Autodesk Inventor part; units mm, degrees
(part 2 of 2)
  line L353 (186.3853, -129.3179) -> (186.3853, -143.3229)
  line L354 (186.3853, -143.3229) -> (172.3803, -143.3229)
  line L355 (172.3803, -143.3229) -> (172.3803, -129.3179)
  line L356 (172.3803, -129.3179) -> (186.3853, -143.3229) construction
  line L357 (186.3853, -129.3179) -> (172.3803, -143.3229) construction
  line L358 (180.9186, -148.2929) -> (194.9236, -148.2929)
  line L359 (194.9236, -148.2929) -> (194.9236, -162.2979)
  line L360 (194.9236, -162.2979) -> (180.9186, -162.2979)
  line L361 (180.9186, -162.2979) -> (180.9186, -148.2929)
  line L362 (180.9186, -148.2929) -> (194.9236, -162.2979) construction
  line L363 (194.9236, -148.2929) -> (180.9186, -162.2979) construction
  line L364 (191.4303, -129.3179) -> (205.4353, -129.3179)
  line L365 (205.4353, -129.3179) -> (205.4353, -143.3229)
  line L366 (205.4353, -143.3229) -> (191.4303, -143.3229)
  line L367 (191.4303, -143.3229) -> (191.4303, -129.3179)
  line L368 (191.4303, -129.3179) -> (205.4353, -143.3229) construction
  line L369 (205.4353, -129.3179) -> (191.4303, -143.3229) construction
  line L370 (200.8283, -110.2679) -> (214.8333, -110.2679)
  line L371 (214.8333, -110.2679) -> (214.8333, -124.2729)
  line L372 (214.8333, -124.2729) -> (200.8283, -124.2729)
  line L373 (200.8283, -124.2729) -> (200.8283, -110.2679)
  line L374 (200.8283, -110.2679) -> (214.8333, -124.2729) construction
  line L375 (214.8333, -110.2679) -> (200.8283, -124.2729) construction
  line L376 (196.0023, -91.2179) -> (210.0073, -91.2179)
  line L377 (210.0073, -91.2179) -> (210.0073, -105.2229)
  line L378 (210.0073, -105.2229) -> (196.0023, -105.2229)
  line L379 (196.0023, -105.2229) -> (196.0023, -91.2179)
  line L380 (196.0023, -91.2179) -> (210.0073, -105.2229) construction
  line L381 (210.0073, -91.2179) -> (196.0023, -105.2229) construction
  line L382 (215.0523, -91.2179) -> (229.0573, -91.2179)
  line L383 (229.0573, -91.2179) -> (229.0573, -105.2229)
  line L384 (229.0573, -105.2229) -> (215.0523, -105.2229)
  line L385 (215.0523, -105.2229) -> (215.0523, -91.2179)
  line L386 (215.0523, -91.2179) -> (229.0573, -105.2229) construction
  line L387 (229.0573, -91.2179) -> (215.0523, -105.2229) construction
  line L388 (219.8783, -110.2679) -> (233.8833, -110.2679)
  line L389 (233.8833, -110.2679) -> (233.8833, -124.2729)
  line L390 (233.8833, -124.2729) -> (219.8783, -124.2729)
  line L391 (219.8783, -124.2729) -> (219.8783, -110.2679)
  line L392 (219.8783, -110.2679) -> (233.8833, -124.2729) construction
  line L393 (233.8833, -110.2679) -> (219.8783, -124.2729) construction
  line L394 (210.4803, -129.3179) -> (224.4853, -129.3179)
  line L395 (224.4853, -129.3179) -> (224.4853, -143.3229)
  line L396 (224.4853, -143.3229) -> (210.4803, -143.3229)
  line L397 (210.4803, -143.3229) -> (210.4803, -129.3179)
  line L398 (210.4803, -129.3179) -> (224.4853, -143.3229) construction
  line L399 (224.4853, -129.3179) -> (210.4803, -143.3229) construction
  line L400 (274.4883, -43.5111) -> (288.4933, -43.5111) construction
  line L401 (288.4933, -43.5111) -> (288.4933, -57.5161) construction
  line L402 (288.4933, -57.5161) -> (274.4883, -57.5161) construction
  line L403 (274.4883, -57.5161) -> (274.4883, -43.5111) construction
  line L404 (274.4883, -43.5111) -> (288.4933, -57.5161) construction
  line L405 (288.4933, -43.5111) -> (274.4883, -57.5161) construction
  line L406 (281.8543, -72.1679) -> (295.8593, -72.1679) construction
  line L407 (295.8593, -72.1679) -> (295.8593, -86.1729) construction
  line L408 (295.8593, -86.1729) -> (281.8543, -86.1729) construction
  line L409 (281.8543, -86.1729) -> (281.8543, -72.1679) construction
  line L410 (281.8543, -72.1679) -> (295.8593, -86.1729) construction
  line L411 (295.8593, -72.1679) -> (281.8543, -86.1729) construction
  line L412 (272.2023, -91.2179) -> (286.2073, -91.2179) construction
  line L413 (286.2073, -91.2179) -> (286.2073, -105.2229) construction
  line L414 (286.2073, -105.2229) -> (272.2023, -105.2229) construction
  line L415 (272.2023, -105.2229) -> (272.2023, -91.2179) construction
  line L416 (272.2023, -91.2179) -> (286.2073, -105.2229) construction
  line L417 (286.2073, -91.2179) -> (272.2023, -105.2229) construction
  line L418 (277.2823, -110.2679) -> (291.2873, -110.2679) construction
  line L419 (291.2873, -110.2679) -> (291.2873, -124.2729) construction
  line L420 (291.2873, -124.2729) -> (277.2823, -124.2729) construction
  line L421 (277.2823, -124.2729) -> (277.2823, -110.2679) construction
  line L422 (277.2823, -110.2679) -> (291.2873, -124.2729) construction
  line L423 (291.2873, -110.2679) -> (277.2823, -124.2729) construction
  line L424 (267.6303, -129.3179) -> (281.6353, -129.3179) construction
  line L425 (281.6353, -129.3179) -> (281.6353, -143.3229) construction
  line L426 (281.6353, -143.3229) -> (267.6303, -143.3229) construction
  line L427 (267.6303, -143.3229) -> (267.6303, -129.3179) construction
  line L428 (267.6303, -129.3179) -> (281.6353, -143.3229) construction
  line L429 (281.6353, -129.3179) -> (267.6303, -143.3229) construction
  line L430 (279.0603, -148.3679) -> (293.0653, -148.3679) construction
  line L431 (293.0653, -148.3679) -> (293.0653, -162.3729) construction
  line L432 (293.0653, -162.3729) -> (279.0603, -162.3729) construction
  line L433 (279.0603, -162.3729) -> (279.0603, -148.3679) construction
  line L434 (279.0603, -148.3679) -> (293.0653, -162.3729) construction
  line L435 (293.0653, -148.3679) -> (279.0603, -162.3729) construction
  line L436 (269.5528, -40) -> (269.5528, -64.842) construction
  line L437 (269.5528, -64.842) -> (279.3318, -64.842) construction
  line L438 (279.3318, -64.842) -> (279.3318, -88.6954) construction
  line L439 (279.3318, -88.6954) -> (269.6798, -88.6954) construction
  line L440 (269.6798, -88.6954) -> (269.6798, -107.7454) construction
  line L441 (269.6798, -107.7454) -> (274.7598, -107.7454) construction
  line L442 (265.1048, -126.7954) -> (265.1048, -151.6615) construction
  line L443 (265.1048, -151.6615) -> (275.5314, -151.6615) construction
  line L444 (275.5314, -151.6615) -> (275.5314, -165) construction
  line L445 (265, -160) -> (275.5314, -160) construction
  line L446 (286.0628, -155.3704) -> (275.5314, -155.3704) construction
  line L447 (265, -160) -> (265, -151.6615) construction
  line L448 (269.0122, -143.3229) -> (269.0122, -151.6615) construction
  line L449 (262.5793, -140.2954) -> (265.1048, -140.2954) construction
  line L450 (265.1048, -140.2954) -> (267.6303, -140.2954) construction
  line L451 (273.1318, -105.2229) -> (273.1318, -107.7454) construction
  line L452 (271.7643, -110.2679) -> (271.7643, -107.7454) construction
  line L453 (267.1573, -99.7852) -> (269.6798, -99.7852) construction
  line L454 (269.6798, -99.7852) -> (272.2023, -99.7852) construction
  line L455 (273.1318, -91.2179) -> (273.1318, -88.6954) construction
  line L456 (273.1318, -88.6954) -> (273.1318, -86.1729) construction
  line L457 (276.8093, -76.5209) -> (279.3318, -76.5209) construction
  line L458 (279.3318, -76.5209) -> (281.8543, -76.5209) construction
  line L459 (276.0401, -72.1679) -> (276.0401, -64.842) construction
  line L460 (276.0401, -64.842) -> (276.0401, -57.5161) construction
  line L461 (264.6173, -51.0859) -> (269.5528, -51.0859) construction
  line L462 (269.5528, -51.0859) -> (274.4883, -51.0859) construction
  line L463 (274.7598, -107.7454) -> (274.7598, -126.7954) construction
  line L464 (272.2373, -121.2454) -> (274.7598, -121.2454) construction
  line L465 (274.7598, -121.2454) -> (277.2823, -121.2454) construction
  line L466 (265.1048, -126.7954) -> (274.7598, -126.7954) construction
  line L467 (270.2657, -124.2729) -> (270.2657, -126.7954) construction
  line L468 (270.2657, -126.7954) -> (270.2657, -129.3179) construction
  line L469 (269.4028, -40) -> (269.4028, -64.992)
  line L470 (269.4028, -64.992) -> (279.1818, -64.992)
  line L471 (279.1818, -64.992) -> (279.1818, -88.5454)
  line L472 (279.1818, -88.5454) -> (269.5298, -88.5454)
  line L473 (269.5298, -88.5454) -> (269.5298, -107.8954)
  line L474 (269.5298, -107.8954) -> (274.6098, -107.8954)
  line L475 (274.6098, -107.8954) -> (274.6098, -126.6454)
  line L476 (274.6098, -126.6454) -> (264.9548, -126.6454)
  line L477 (264.9548, -126.6454) -> (264.9548, -151.8115)
  line L478 (264.9548, -151.8115) -> (275.3814, -151.8115)
  line L479 (275.3814, -151.8115) -> (275.3814, -165)
  line L480 (275.3814, -165) -> (40, -165)
  line L481 (40, -165) -> (40, -40)
  line L482 (40, -40) -> (269.4028, -40)
  circle A409 centre (45, -127) radius 3.25
  circle A410 centre (45, -64.8616) radius 3.25
  line L483 (172.0148, -58.6601) -> (214.7648, -58.6601)
  line L484 (214.7648, -58.6601) -> (214.7648, -65.1601)
  line L485 (214.7648, -65.1601) -> (172.0148, -65.1601)
  line L486 (172.0148, -65.1601) -> (172.0148, -58.6601)
  circle A411 centre (155, -64.8616) radius 3.25
  circle A412 centre (265, -64.8616) radius 3.25
  point P0 (0, 0)
  point P1 (274.7598, -117.2704)
  point P2 (46.7679, -124.2729)
  point P3 (46.1423, -123.9574)
  dimension "d0" = 6.5
  dimension "d1" = 14.005
  dimension "d2" = 14.005
  dimension "d3" = 14.005
  dimension "d4" = 14.005
  dimension "d5" = 14.005
  dimension "d6" = 14.005
  dimension "d7" = 14.005
  dimension "d8" = 14.005
  dimension "d9" = 14.005
  dimension "d10" = 14.005
  dimension "d11" = 14.005
  dimension "d12" = 14.005
  dimension "d13" = 14.005
  dimension "d14" = 14.005
  dimension "d15" = 14.005
  dimension "d16" = 14.005
  dimension "d17" = 14.005
  dimension "d18" = 14.005
  dimension "d19" = 14.005
  dimension "d20" = 14.005
  dimension "d21" = 14.005
  dimension "d22" = 14.005
  dimension "d23" = 14.005
  dimension "d24" = 14.005
  dimension "d25" = 14.005
  dimension "d26" = 14.005
  dimension "d27" = 14.005
  dimension "d28" = 14.005
  dimension "d29" = 14.005
  dimension "d30" = 14.005
  dimension "d31" = 14.005
  dimension "d32" = 14.005
  dimension "d33" = 14.005
  dimension "d34" = 14.005
  dimension "d35" = 14.005
  dimension "d36" = 14.005
  dimension "d37" = 14.005
  dimension "d38" = 14.005
  dimension "d39" = 14.005
  dimension "d40" = 14.005
  dimension "d41" = 14.005
  dimension "d42" = 14.005
  dimension "d43" = 14.005
  dimension "d44" = 14.005
  dimension "d45" = 14.005
  dimension "d46" = 14.005
  dimension "d47" = 14.005
  dimension "d48" = 14.005
  dimension "d49" = 14.005
  dimension "d50" = 14.005
  dimension "d51" = 14.005
  dimension "d52" = 14.005
  dimension "d53" = 14.005
  dimension "d54" = 14.005
  dimension "d55" = 14.005
  dimension "d56" = 14.005
  dimension "d57" = 14.005
  dimension "d58" = 14.005
  dimension "d59" = 14.005
  dimension "d60" = 14.005
  dimension "d61" = 14.005
  dimension "d62" = 14.005
  dimension "d63" = 14.005
  constraints: 870 end point, 132 parallel, 129 midpoint, 92 perpendicular, 67 horizontal, 47 point on line, 11 equal length, 7 coincident, 6 centre point, 5 equal radius, 3 collinear, 2 vertical
  measures "d0" diameter of A407
  measures "d1" distance of L54.end L53.end
  measures "d2" distance of L53.end L52.end
  measures "d3" distance of L59.end L60.end
  measures "d4" distance of L58.end L59.end
  measures "d5" distance of L65.end L66.end
  measures "d6" distance of L64.end L65.end
  measures "d7" distance of L71.end L72.end
  measures "d8" distance of L70.end L71.end
  measures "d9" distance of L77.end L78.end
  measures "d10" distance of L76.end L77.end
  measures "d11" distance of L83.end L84.end
  measures "d12" distance of L82.end L83.end
  measures "d13" distance of L89.end L90.end
  measures "d14" distance of L88.end L89.end
  measures "d15" distance of L95.end L96.end
  measures "d16" distance of L94.end L95.end
  measures "d17" distance of L101.end L102.end
  measures "d18" distance of L100.end L101.end
  measures "d19" distance of L107.end L108.end
  measures "d20" distance of L106.end L107.end
  measures "d21" distance of L113.end L114.end
  measures "d22" distance of L112.end L113.end
  measures "d23" distance of L119.end L120.end
  measures "d24" distance of L118.end L119.end
  measures "d25" distance of L125.end L126.end
  measures "d26" distance of L124.end L125.end
  measures "d27" distance of L131.end L132.end
  measures "d28" distance of L130.end L131.end
  measures "d29" distance of L137.end L138.end
  measures "d30" distance of L136.end L137.end
  measures "d31" distance of L143.end L144.end
  measures "d32" distance of L142.end L143.end
  measures "d33" distance of L149.end L150.end
  measures "d34" distance of L148.end L149.end
  measures "d35" distance of L155.end L156.end
  measures "d36" distance of L154.end L155.end
  measures "d37" distance of L161.end L162.end
  measures "d38" distance of L160.end L161.end
  measures "d39" distance of L167.end L168.end
  measures "d40" distance of L166.end L167.end
  measures "d41" distance of L173.end L174.end
  measures "d42" distance of L172.end L173.end
  measures "d43" distance of L179.end L180.end
  measures "d44" distance of L178.end L179.end
  measures "d45" distance of L185.end L186.end
  measures "d46" distance of L184.end L185.end
  measures "d47" distance of L191.end L192.end
  measures "d48" distance of L190.end L191.end
  measures "d49" distance of L197.end L198.end
  measures "d50" distance of L196.end L197.end
  measures "d51" distance of L203.end L204.end
  measures "d52" distance of L202.end L203.end
  measures "d53" distance of L209.end L210.end
  measures "d54" distance of L208.end L209.end
  measures "d55" distance of L215.end L216.end
  measures "d56" distance of L214.end L215.end
  measures "d57" distance of L221.end L222.end
  measures "d58" distance of L220.end L221.end
  measures "d59" distance of L227.end L228.end
  measures "d60" distance of L226.end L227.end
  measures "d61" distance of L233.end L234.end
  measures "d62" distance of L232.end L233.end
  measures "d63" distance of L239.end L240.end
extrude "Extrusion3" add sketch "Sketch1" along normal blind 0.5
sketch "Sketch3" plane through (0, 0, 0.5) normal (0, 0, 1) x (1, 0, 0)
  line L0 (40, -40) -> (40, -165) projected
  line L1 (40, -165) -> (275.3814, -165) projected
  line L2 (275.3814, -165) -> (275.3814, -151.8115) projected
  line L3 (275.3814, -151.8115) -> (264.9548, -151.8115) projected
  line L4 (264.9548, -151.8115) -> (264.9548, -126.6454) projected
  line L5 (264.9548, -126.6454) -> (274.6098, -126.6454) projected
  line L6 (274.6098, -126.6454) -> (274.6098, -107.8954) projected
  line L7 (274.6098, -107.8954) -> (269.5298, -107.8954) projected
  line L8 (269.5298, -107.8954) -> (269.5298, -88.5454) projected
  line L9 (269.5298, -88.5454) -> (279.1818, -88.5454) projected
  line L10 (279.1818, -88.5454) -> (279.1818, -64.992) projected
  line L11 (279.1818, -64.992) -> (269.4028, -64.992) projected
  line L12 (269.4028, -64.992) -> (269.4028, -40) projected
  line L13 (269.4028, -40) -> (40, -40) projected
  circle A0 centre (155, -160) radius 3.25 projected
  circle A1 centre (265, -160) radius 3.25 projected
  circle A2 centre (45, -64.8616) radius 3.25 projected
  circle A3 centre (155, -64.8616) radius 3.25 projected
  circle A4 centre (265, -64.8616) radius 3.25 projected
  line L14 (172.0148, -58.6601) -> (214.7648, -58.6601) projected
  line L15 (214.7648, -58.6601) -> (214.7648, -65.1601) projected
  line L16 (214.7648, -65.1601) -> (172.0148, -65.1601) projected
  line L17 (172.0148, -65.1601) -> (172.0148, -58.6601) projected
  line L18 (210.4803, -129.3179) -> (224.4853, -129.3179) projected
  line L19 (224.4853, -129.3179) -> (224.4853, -143.3229) projected
  line L20 (224.4853, -143.3229) -> (210.4803, -143.3229) projected
  line L21 (210.4803, -143.3229) -> (210.4803, -129.3179) projected
  line L22 (219.8783, -110.2679) -> (233.8833, -110.2679) projected
  line L23 (233.8833, -110.2679) -> (233.8833, -124.2729) projected
  line L24 (233.8833, -124.2729) -> (219.8783, -124.2729) projected
  line L25 (219.8783, -124.2729) -> (219.8783, -110.2679) projected
  line L26 (215.0523, -91.2179) -> (229.0573, -91.2179) projected
  line L27 (229.0573, -91.2179) -> (229.0573, -105.2229) projected
  line L28 (229.0573, -105.2229) -> (215.0523, -105.2229) projected
  line L29 (215.0523, -105.2229) -> (215.0523, -91.2179) projected
  line L30 (196.0023, -91.2179) -> (210.0073, -91.2179) projected
  line L31 (210.0073, -91.2179) -> (210.0073, -105.2229) projected
  line L32 (210.0073, -105.2229) -> (196.0023, -105.2229) projected
  line L33 (196.0023, -105.2229) -> (196.0023, -91.2179) projected
  line L34 (200.8283, -110.2679) -> (214.8333, -110.2679) projected
  line L35 (214.8333, -110.2679) -> (214.8333, -124.2729) projected
  line L36 (214.8333, -124.2729) -> (200.8283, -124.2729) projected
  line L37 (200.8283, -124.2729) -> (200.8283, -110.2679) projected
  line L38 (191.4303, -129.3179) -> (205.4353, -129.3179) projected
  line L39 (205.4353, -129.3179) -> (205.4353, -143.3229) projected
  line L40 (205.4353, -143.3229) -> (191.4303, -143.3229) projected
  line L41 (191.4303, -143.3229) -> (191.4303, -129.3179) projected
  line L42 (180.9186, -148.2929) -> (194.9236, -148.2929) projected
  line L43 (194.9236, -148.2929) -> (194.9236, -162.2979) projected
  line L44 (194.9236, -162.2979) -> (180.9186, -162.2979) projected
  line L45 (180.9186, -162.2979) -> (180.9186, -148.2929) projected
  line L46 (172.3803, -129.3179) -> (186.3853, -129.3179) projected
  line L47 (186.3853, -129.3179) -> (186.3853, -143.3229) projected
  line L48 (186.3853, -143.3229) -> (172.3803, -143.3229) projected
  line L49 (172.3803, -143.3229) -> (172.3803, -129.3179) projected
  line L50 (181.7783, -110.2679) -> (195.7833, -110.2679) projected
  line L51 (195.7833, -110.2679) -> (195.7833, -124.2729) projected
  line L52 (195.7833, -124.2729) -> (181.7783, -124.2729) projected
  line L53 (181.7783, -124.2729) -> (181.7783, -110.2679) projected
  line L54 (176.9523, -91.2179) -> (190.9573, -91.2179) projected
  line L55 (190.9573, -91.2179) -> (190.9573, -105.2229) projected
  line L56 (190.9573, -105.2229) -> (176.9523, -105.2229) projected
  line L57 (176.9523, -105.2229) -> (176.9523, -91.2179) projected
  line L58 (162.7283, -110.2679) -> (176.7333, -110.2679) projected
  line L59 (176.7333, -110.2679) -> (176.7333, -124.2729) projected
  line L60 (176.7333, -124.2729) -> (162.7283, -124.2729) projected
  line L61 (162.7283, -124.2729) -> (162.7283, -110.2679) projected
  line L62 (157.9023, -91.2967) -> (171.9073, -91.2967) projected
  line L63 (171.9073, -91.2967) -> (171.9073, -105.3017) projected
  line L64 (171.9073, -105.3017) -> (157.9023, -105.3017) projected
  line L65 (157.9023, -105.3017) -> (157.9023, -91.2967) projected
  line L66 (153.3303, -129.3179) -> (167.3353, -129.3179) projected
  line L67 (167.3353, -129.3179) -> (167.3353, -143.3229) projected
  line L68 (167.3353, -143.3229) -> (153.3303, -143.3229) projected
  line L69 (153.3303, -143.3229) -> (153.3303, -129.3179) projected
  line L70 (134.2803, -129.3179) -> (148.2853, -129.3179) projected
  line L71 (148.2853, -129.3179) -> (148.2853, -143.3229) projected
  line L72 (148.2853, -143.3229) -> (134.2803, -143.3229) projected
  line L73 (134.2803, -143.3229) -> (134.2803, -129.3179) projected
  line L74 (143.6783, -110.2679) -> (157.6833, -110.2679) projected
  line L75 (157.6833, -110.2679) -> (157.6833, -124.2729) projected
  line L76 (157.6833, -124.2729) -> (143.6783, -124.2729) projected
  line L77 (143.6783, -124.2729) -> (143.6783, -110.2679) projected
  line L78 (138.8523, -91.2179) -> (152.8573, -91.2179) projected
  line L79 (152.8573, -91.2179) -> (152.8573, -105.2229) projected
  line L80 (152.8573, -105.2229) -> (138.8523, -105.2229) projected
  line L81 (138.8523, -105.2229) -> (138.8523, -91.2179) projected
  line L82 (119.8023, -91.2179) -> (133.8073, -91.2179) projected
  line L83 (133.8073, -91.2179) -> (133.8073, -105.2229) projected
  line L84 (133.8073, -105.2229) -> (119.8023, -105.2229) projected
  line L85 (119.8023, -105.2229) -> (119.8023, -91.2179) projected
  line L86 (124.6283, -110.2679) -> (138.6333, -110.2679) projected
  line L87 (138.6333, -110.2679) -> (138.6333, -124.2729) projected
  line L88 (138.6333, -124.2729) -> (124.6283, -124.2729) projected
  line L89 (124.6283, -124.2729) -> (124.6283, -110.2679) projected
  line L90 (115.2303, -129.3179) -> (129.2353, -129.3179) projected
  line L91 (129.2353, -129.3179) -> (129.2353, -143.3229) projected
  line L92 (129.2353, -143.3229) -> (115.2303, -143.3229) projected
  line L93 (115.2303, -143.3229) -> (115.2303, -129.3179) projected
  line L94 (96.1803, -129.3179) -> (110.1853, -129.3179) projected
  line L95 (110.1853, -129.3179) -> (110.1853, -143.3229) projected
  line L96 (110.1853, -143.3229) -> (96.1803, -143.3229) projected
  line L97 (96.1803, -143.3229) -> (96.1803, -129.3179) projected
  line L98 (105.5783, -110.2679) -> (119.5833, -110.2679) projected
  line L99 (119.5833, -110.2679) -> (119.5833, -124.2729) projected
  line L100 (119.5833, -124.2729) -> (105.5783, -124.2729) projected
  line L101 (105.5783, -124.2729) -> (105.5783, -110.2679) projected
  line L102 (100.7523, -91.2179) -> (114.7573, -91.2179) projected
  line L103 (114.7573, -91.2179) -> (114.7573, -105.2229) projected
  line L104 (114.7573, -105.2229) -> (100.7523, -105.2229) projected
  line L105 (100.7523, -105.2229) -> (100.7523, -91.2179) projected
  line L106 (86.5283, -110.2679) -> (100.5333, -110.2679) projected
  line L107 (100.5333, -110.2679) -> (100.5333, -124.2729) projected
  line L108 (100.5333, -124.2729) -> (86.5283, -124.2729) projected
  line L109 (86.5283, -124.2729) -> (86.5283, -110.2679) projected
  line L110 (77.1303, -129.3179) -> (91.1353, -129.3179) projected
  line L111 (91.1353, -129.3179) -> (91.1353, -143.3229) projected
  line L112 (91.1353, -143.3229) -> (77.1303, -143.3229) projected
  line L113 (77.1303, -143.3229) -> (77.1303, -129.3179) projected
  line L114 (83.7343, -148.3679) -> (97.7393, -148.3679) projected
  line L115 (97.7393, -148.3679) -> (97.7393, -162.3729) projected
  line L116 (97.7393, -162.3729) -> (83.7343, -162.3729) projected
  line L117 (83.7343, -162.3729) -> (83.7343, -148.3679) projected
  line L118 (59.8583, -148.3679) -> (73.8633, -148.3679) projected
  line L119 (73.8633, -148.3679) -> (73.8633, -162.3729) projected
  line L120 (73.8633, -162.3729) -> (59.8583, -162.3729) projected
  line L121 (59.8583, -162.3729) -> (59.8583, -148.3679) projected
  line L122 (50.9683, -129.3179) -> (64.9733, -129.3179) projected
  line L123 (64.9733, -129.3179) -> (64.9733, -143.3229) projected
  line L124 (64.9733, -143.3229) -> (50.9683, -143.3229) projected
  line L125 (50.9683, -143.3229) -> (50.9683, -129.3179) projected
  line L126 (67.4783, -110.2679) -> (81.4833, -110.2679) projected
  line L127 (81.4833, -110.2679) -> (81.4833, -124.2729) projected
  line L128 (81.4833, -124.2729) -> (67.4783, -124.2729) projected
  line L129 (67.4783, -124.2729) -> (67.4783, -110.2679) projected
  line L130 (81.7023, -91.2179) -> (95.7073, -91.2179) projected
  line L131 (95.7073, -91.2179) -> (95.7073, -105.2229) projected
  line L132 (95.7073, -105.2229) -> (81.7023, -105.2229) projected
  line L133 (81.7023, -105.2229) -> (81.7023, -91.2179) projected
  line L134 (53.2543, -91.2179) -> (67.2593, -91.2179) projected
  line L135 (67.2593, -91.2179) -> (67.2593, -105.2229) projected
  line L136 (67.2593, -105.2229) -> (53.2543, -105.2229) projected
  line L137 (53.2543, -105.2229) -> (53.2543, -91.2179) projected
  line L138 (48.5263, -72.1679) -> (62.5313, -72.1679) projected
  line L139 (62.5313, -72.1679) -> (62.5313, -86.1729) projected
  line L140 (62.5313, -86.1729) -> (48.5263, -86.1729) projected
  line L141 (48.5263, -86.1729) -> (48.5263, -72.1679) projected
  line L142 (72.3043, -72.1679) -> (86.3093, -72.1679) projected
  line L143 (86.3093, -72.1679) -> (86.3093, -86.1729) projected
  line L144 (86.3093, -86.1729) -> (72.3043, -86.1729) projected
  line L145 (72.3043, -86.1729) -> (72.3043, -72.1679) projected
  line L146 (91.3543, -72.1679) -> (105.3593, -72.1679) projected
  line L147 (105.3593, -72.1679) -> (105.3593, -86.1729) projected
  line L148 (105.3593, -86.1729) -> (91.3543, -86.1729) projected
  line L149 (91.3543, -86.1729) -> (91.3543, -72.1679) projected
  line L150 (110.4043, -72.1679) -> (124.4093, -72.1679) projected
  line L151 (124.4093, -72.1679) -> (124.4093, -86.1729) projected
  line L152 (124.4093, -86.1729) -> (110.4043, -86.1729) projected
  line L153 (110.4043, -86.1729) -> (110.4043, -72.1679) projected
  line L154 (129.4543, -72.1679) -> (143.4593, -72.1679) projected
  line L155 (143.4593, -72.1679) -> (143.4593, -86.1729) projected
  line L156 (143.4593, -86.1729) -> (129.4543, -86.1729) projected
  line L157 (129.4543, -86.1729) -> (129.4543, -72.1679) projected
  line L158 (148.5043, -72.1679) -> (162.5093, -72.1679) projected
  line L159 (162.5093, -72.1679) -> (162.5093, -86.1729) projected
  line L160 (162.5093, -86.1729) -> (148.5043, -86.1729) projected
  line L161 (148.5043, -86.1729) -> (148.5043, -72.1679) projected
  line L162 (167.5543, -72.1679) -> (181.5593, -72.1679) projected
  line L163 (181.5593, -72.1679) -> (181.5593, -86.1729) projected
  line L164 (181.5593, -86.1729) -> (167.5543, -86.1729) projected
  line L165 (167.5543, -86.1729) -> (167.5543, -72.1679) projected
  line L166 (186.6043, -72.1679) -> (200.6093, -72.1679) projected
  line L167 (200.6093, -72.1679) -> (200.6093, -86.1729) projected
  line L168 (200.6093, -86.1729) -> (186.6043, -86.1729) projected
  line L169 (186.6043, -86.1729) -> (186.6043, -72.1679) projected
  line L170 (205.6543, -72.1679) -> (219.6593, -72.1679) projected
  line L171 (219.6593, -72.1679) -> (219.6593, -86.1729) projected
  line L172 (219.6593, -86.1729) -> (205.6543, -86.1729) projected
  line L173 (205.6543, -86.1729) -> (205.6543, -72.1679) projected
  line L174 (224.7043, -72.1679) -> (238.7093, -72.1679) projected
  line L175 (238.7093, -72.1679) -> (238.7093, -86.1729) projected
  line L176 (238.7093, -86.1729) -> (224.7043, -86.1729) projected
  line L177 (224.7043, -86.1729) -> (224.7043, -72.1679) projected
  line L178 (243.7543, -72.1679) -> (257.7593, -72.1679) projected
  line L179 (257.7593, -72.1679) -> (257.7593, -86.1729) projected
  line L180 (257.7593, -86.1729) -> (243.7543, -86.1729) projected
  line L181 (243.7543, -86.1729) -> (243.7543, -72.1679) projected
  line L182 (234.1023, -91.2179) -> (248.1073, -91.2179) projected
  line L183 (248.1073, -91.2179) -> (248.1073, -105.2229) projected
  line L184 (248.1073, -105.2229) -> (234.1023, -105.2229) projected
  line L185 (234.1023, -105.2229) -> (234.1023, -91.2179) projected
  line L186 (238.9283, -110.2679) -> (252.9333, -110.2679) projected
  line L187 (252.9333, -110.2679) -> (252.9333, -124.2729) projected
  line L188 (252.9333, -124.2729) -> (238.9283, -124.2729) projected
  line L189 (238.9283, -124.2729) -> (238.9283, -110.2679) projected
  line L190 (229.5343, -129.3199) -> (243.5393, -129.3199) projected
  line L191 (243.5393, -129.3199) -> (243.5393, -143.3249) projected
  line L192 (243.5393, -143.3249) -> (229.5343, -143.3249) projected
  line L193 (229.5343, -143.3249) -> (229.5343, -129.3199) projected
  line L194 (248.5743, -129.3399) -> (262.5793, -129.3399) projected
  line L195 (262.5793, -129.3399) -> (262.5793, -143.3449) projected
  line L196 (262.5793, -143.3449) -> (248.5743, -143.3449) projected
  line L197 (248.5743, -143.3449) -> (248.5743, -129.3399) projected
  line L198 (258.2323, -110.2679) -> (272.2373, -110.2679) projected
  line L199 (272.2373, -110.2679) -> (272.2373, -124.2729) projected
  line L200 (272.2373, -124.2729) -> (258.2323, -124.2729) projected
  line L201 (258.2323, -124.2729) -> (258.2323, -110.2679) projected
  line L202 (253.1523, -91.2179) -> (267.1573, -91.2179) projected
  line L203 (267.1573, -91.2179) -> (267.1573, -105.2229) projected
  line L204 (267.1573, -105.2229) -> (253.1523, -105.2229) projected
  line L205 (253.1523, -105.2229) -> (253.1523, -91.2179) projected
  line L206 (262.8043, -72.1679) -> (276.8093, -72.1679) projected
  line L207 (276.8093, -72.1679) -> (276.8093, -86.1729) projected
  line L208 (276.8093, -86.1729) -> (262.8043, -86.1729) projected
  line L209 (262.8043, -86.1729) -> (262.8043, -72.1679) projected
  line L210 (250.6123, -43.5111) -> (264.6173, -43.5111) projected
  line L211 (264.6173, -43.5111) -> (264.6173, -57.5161) projected
  line L212 (264.6173, -57.5161) -> (250.6123, -57.5161) projected
  line L213 (250.6123, -57.5161) -> (250.6123, -43.5111) projected
  line L214 (226.7363, -43.5111) -> (240.7413, -43.5111) projected
  line L215 (240.7413, -43.5111) -> (240.7413, -57.5161) projected
  line L216 (240.7413, -57.5161) -> (226.7363, -57.5161) projected
  line L217 (226.7363, -57.5161) -> (226.7363, -43.5111) projected
  line L218 (202.8543, -43.5111) -> (216.8593, -43.5111) projected
  line L219 (216.8593, -43.5111) -> (216.8593, -57.5161) projected
  line L220 (216.8593, -57.5161) -> (202.8543, -57.5161) projected
  line L221 (202.8543, -57.5161) -> (202.8543, -43.5111) projected
  line L222 (170.3483, -43.5111) -> (184.3533, -43.5111) projected
  line L223 (184.3533, -43.5111) -> (184.3533, -57.5161) projected
  line L224 (184.3533, -57.5161) -> (170.3483, -57.5161) projected
  line L225 (170.3483, -57.5161) -> (170.3483, -43.5111) projected
  line L226 (146.4723, -43.5111) -> (160.4773, -43.5111) projected
  line L227 (160.4773, -43.5111) -> (160.4773, -57.5161) projected
  line L228 (160.4773, -57.5161) -> (146.4723, -57.5161) projected
  line L229 (146.4723, -57.5161) -> (146.4723, -43.5111) projected
  line L230 (122.5963, -43.5391) -> (136.6013, -43.5391) projected
  line L231 (136.6013, -43.5391) -> (136.6013, -57.5441) projected
  line L232 (136.6013, -57.5441) -> (122.5963, -57.5441) projected
  line L233 (122.5963, -57.5441) -> (122.5963, -43.5391) projected
  line L234 (98.7203, -43.5111) -> (112.7253, -43.5111) projected
  line L235 (112.7253, -43.5111) -> (112.7253, -57.5161) projected
  line L236 (112.7253, -57.5161) -> (98.7203, -57.5161) projected
  line L237 (98.7203, -57.5161) -> (98.7203, -43.5111) projected
  line L238 (74.9047, -43.3959) -> (88.9097, -43.3959) projected
  line L239 (88.9097, -43.3959) -> (88.9097, -57.4009) projected
  line L240 (88.9097, -57.4009) -> (74.9047, -57.4009) projected
  line L241 (74.9047, -57.4009) -> (74.9047, -43.3959) projected
  line L242 (43.8563, -57.6141) -> (43.8563, -43.6091) projected
  line L243 (43.8563, -43.6091) -> (57.8613, -43.6091) projected
  line L244 (57.8613, -43.6091) -> (57.8613, -57.6141) projected
  line L245 (57.8613, -57.6141) -> (43.8563, -57.6141) projected
  line L246 (60.1473, -110.2679) -> (60.1473, -124.2729) projected
  line L247 (60.1473, -124.2729) -> (46.7679, -124.2729) projected
  arc A5 (46.1423, -123.9574) -> (46.7679, -124.2729) centre (45, -127) ccw projected
  line L248 (46.1423, -123.9574) -> (46.1423, -110.2679) projected
  line L249 (46.1423, -110.2679) -> (60.1473, -110.2679) projected
  line L250 (40, -40) -> (60.3613, -40)
  line L251 (60.3613, -40) -> (60.3613, -60.1141)
  line L252 (60.3613, -60.1141) -> (40, -60.1141)
  line L253 (40, -60.1141) -> (40, -40)
  line L254 (70.7047, -40) -> (188.5533, -40)
  line L255 (188.5533, -40) -> (188.5533, -58.6601)
  line L256 (172.0148, -60.1141) -> (70.7047, -60.1141)
  line L257 (70.7047, -60.1141) -> (70.7047, -40)
  line L258 (172.0148, -60.1141) -> (172.0148, -58.6601)
  line L259 (172.0148, -58.6601) -> (214.7648, -58.6601) projected
  line L260 (172.0148, -58.6601) -> (188.5533, -58.6601)
  line L261 (198.6543, -40) -> (269.4028, -40)
  line L262 (269.4028, -40) -> (269.4028, -60.1141)
  line L263 (269.4028, -60.1141) -> (214.7648, -60.1141)
  line L264 (198.6543, -58.6601) -> (198.6543, -40)
  line L265 (198.6543, -58.6601) -> (214.7648, -58.6601)
  line L266 (214.7648, -58.6601) -> (214.7648, -60.1141)
  line L267 (40, -69.6679) -> (279.1818, -69.6679)
  point P0 (0, 0)
  dimension "d152" = 2.5
  dimension "d153" = 2.5
  dimension "d154" = 4.2
  dimension "d155" = 4.2
  dimension "d156" = 4.2
  dimension "d157" = 2.5
  constraints: 34 end point, 9 point on line, 7 parallel, 4 perpendicular, 3 collinear, 3 horizontal
  measures "d152" distance between parallel lines of L251 L244
  measures "d153" distance between parallel lines of L252 L245
  measures "d154" distance between parallel lines of L241 L257
  measures "d155" distance between parallel lines of L255 L223
  measures "d156" distance between parallel lines of L221 L264
  measures "d157" distance between parallel lines of L267 L138
extrude "Extrusion4" add sketch "Sketch3" along normal blind 2.5 contours L13 L251 L252 L0 | L267 L10 L9 L8 L7 L6 L5 L4 L3 L2 L1 L0 | L13 L255 L14 L17 L256 L257 | L13 L12 L263 L15 L14 L264
equation "\"d1\" = sd"
equation "\"d2\" = sd"
equation "\"d3\" = sd"
equation "\"d4\" = sd"
equation "\"d5\" = sd"
equation "\"d6\" = sd"
equation "\"d7\" = sd"
equation "\"d8\" = sd"
equation "\"d9\" = sd"
equation "\"d10\" = sd"
equation "\"d11\" = sd"
equation "\"d12\" = sd"
equation "\"d13\" = sd"
equation "\"d14\" = sd"
equation "\"d15\" = sd"
equation "\"d16\" = sd"
equation "\"d17\" = sd"
equation "\"d18\" = sd"
equation "\"d19\" = sd"
equation "\"d20\" = sd"
equation "\"d21\" = sd"
equation "\"d22\" = sd"
equation "\"d23\" = sd"
equation "\"d24\" = sd"
equation "\"d25\" = sd"
equation "\"d26\" = sd"
equation "\"d27\" = sd"
equation "\"d28\" = sd"
equation "\"d29\" = sd"
equation "\"d30\" = sd"
equation "\"d31\" = sd"
equation "\"d32\" = sd"
equation "\"d33\" = sd"
equation "\"d34\" = sd"
equation "\"d35\" = sd"
equation "\"d36\" = sd"
equation "\"d37\" = sd"
equation "\"d38\" = sd"
equation "\"d39\" = sd"
equation "\"d40\" = sd"
equation "\"d41\" = sd"
equation "\"d42\" = sd"
equation "\"d43\" = sd"
equation "\"d44\" = sd"
equation "\"d45\" = sd"
equation "\"d46\" = sd"
equation "\"d47\" = sd"
equation "\"d48\" = sd"
equation "\"d49\" = sd"
equation "\"d50\" = sd"
equation "\"d51\" = sd"
equation "\"d52\" = sd"
equation "\"d53\" = sd"
equation "\"d54\" = sd"
equation "\"d55\" = sd"
equation "\"d56\" = sd"
equation "\"d57\" = sd"
equation "\"d58\" = sd"
equation "\"d59\" = sd"
equation "\"d60\" = sd"
equation "\"d61\" = sd"
equation "\"d62\" = sd"
equation "\"d63\" = sd"
equation "\"sd\" = 14.005"
equation "\"d64\" = sd"
equation "\"d65\" = sd"
equation "\"d66\" = sd"
equation "\"d67\" = sd"
equation "\"d68\" = sd"
equation "\"d69\" = sd"
equation "\"d70\" = sd"
equation "\"d71\" = sd"
equation "\"d72\" = sd"
equation "\"d73\" = sd"
equation "\"d74\" = sd"
equation "\"d75\" = sd"
equation "\"d76\" = sd"
equation "\"d77\" = sd"
equation "\"d78\" = sd"
equation "\"d79\" = sd"
equation "\"d80\" = sd"
equation "\"d81\" = sd"
equation "\"d82\" = sd"
equation "\"d83\" = sd"
equation "\"d84\" = sd"
equation "\"d85\" = sd"
equation "\"d86\" = sd"
equation "\"d87\" = sd"
equation "\"d88\" = sd"
equation "\"d89\" = sd"
equation "\"d90\" = sd"
equation "\"d91\" = sd"
equation "\"d92\" = sd"
equation "\"d93\" = sd"
equation "\"d94\" = sd"
equation "\"d95\" = sd"
equation "\"d96\" = sd"
equation "\"d97\" = sd"
equation "\"d98\" = sd"
equation "\"d99\" = sd"
equation "\"d100\" = sd"
equation "\"d101\" = sd"
equation "\"d102\" = sd"
equation "\"d103\" = sd"
equation "\"d104\" = sd"
equation "\"d105\" = sd"
equation "\"d106\" = sd"
equation "\"d107\" = sd"
equation "\"d108\" = sd"
equation "\"d109\" = sd"
equation "\"d110\" = sd"
equation "\"d111\" = sd"
equation "\"d112\" = sd"
equation "\"d113\" = sd"
equation "\"d114\" = sd"
equation "\"d115\" = sd"
equation "\"d116\" = sd"
equation "\"d117\" = sd"
equation "\"d118\" = sd"
body "Solid3"
